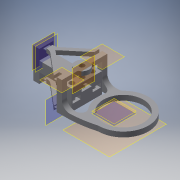
# Autodesk Inventor part: 20_Z-Focus
Saved by Autodesk Inventor 2016 (Build 200138000, 138)
## iProperties
Created: 2016-09-11
Part Number: 20_Z-Focus
Material: Generisch
Document SubType Name: Modeling
Designer: Bene
Density: 1 g/cm^3
Appearance: Vorgabe
Mass: 18.9967 g
Surface Area: 116.758 cm^2
Volume: 18.9967 cm^3
Author: Bene
Autodesk Inventor part; units mm, degrees
ref_plane "YZ Plane" through (0, 0, 0) normal (1, 0, 0) x (0, 1, 0)
ref_plane "XZ Plane" through (0, 0, 0) normal (0, 1, 0) x (-1, 0, 0)
ref_plane "XY Plane" through (0, 0, 0) normal (0, 0, 1) x (1, 0, 0)
ref_plane "Arbeitsebene1" through (0, 0, 0) normal (0, 0, 1) x (1, 0, 0)
ref_plane "Arbeitsebene4" through (-19.17, -30.8266, 13.7758) normal (0, 0, -1) x (-1, 0, 0)
sketch "Skizze3" plane through (-19.17, -30.8266, 13.7758) normal (0, 0, -1) x (-1, 0, 0)
  line L0 (-21.1671, -34.6734) -> (18.8329, -34.6734) construction
  line L1 (23.0052, -34.6734) -> (20.8531, -34.6734) construction
  line L2 (20.8531, -34.6734) -> (20.8531, -31.1843) construction
  line L3 (20.8531, -31.1843) -> (23.0052, -31.1843) construction
  line L4 (23.0052, -31.1843) -> (23.0052, -34.6734) construction
  circle A0 centre (-1.1671, 0.3266) radius 17.5 construction
  line L5 (22.5809, -17.1574) -> (29.5806, -17.1574) construction
  line L6 (29.5806, -17.1574) -> (29.5806, -22.1574) construction
  line L7 (29.5806, -22.1574) -> (28.8232, -22.1574) construction
  line L8 (-0.4194, -22.1574) -> (-0.4194, -17.1574) construction
  line L9 (-0.4194, -22.1574) -> (-21.1671, -22.1574) construction
  line L10 (-21.1671, -22.1574) -> (-21.1671, -17.1574) construction
  line L11 (-21.1671, -17.1574) -> (-0.4194, -17.1574) construction
  line L12 (-0.4194, -17.1574) -> (-0.4194, -22.1574) construction
  line L13 (-21.1671, -17.1574) -> (-17.1671, -17.1574) construction
  line L14 (-17.1671, -17.1574) -> (-17.1671, 0.3266) construction
  line L15 (-17.1671, 0.3266) -> (-21.1671, 0.3266) construction
  line L16 (-21.1671, 0.3266) -> (-21.1671, -17.1574) construction
  line L17 (22.5809, -17.1574) -> (18.5809, -17.1574) construction
  line L18 (18.5809, -10.4487) -> (18.5809, 0.3266) construction
  line L19 (18.5809, 0.3266) -> (22.5809, 0.3266) construction
  line L20 (22.5809, 0.3266) -> (22.5809, -17.1574) construction
  arc A1 (18.5809, -10.4487) -> (-0.4194, -22.1574) centre (-1.1671, 0.3266) ccw construction
  arc A2 (-18.6671, 0.3266) -> (-0.4194, -17.1574) centre (-1.1671, 0.3266) ccw construction
  line L21 (-18.6671, 0.3266) -> (-23.6635, 0.3266) construction
  line L22 (29.5806, -22.1574) -> (-1.9147, -22.1574) construction
  line L23 (29.5806, -17.1574) -> (29.5806, -22.1574)
  arc A3 (-18.6671, 0.3266) -> (16.3329, 0.3266) centre (-1.1671, 0.3266) ccw construction
  line L24 (16.3329, 0.3266) -> (21.3294, 0.3266) construction
  line L25 (-18.6671, 0.3266) -> (-23.6635, 0.3266) construction
  arc A4 (-23.6635, 0.3266) -> (-0.4194, -22.1574) centre (-1.1671, 0.3266) ccw construction
  arc A5 (12.9892, -17.1574) -> (21.3294, 0.3266) centre (-1.1671, 0.3266) ccw construction
  line L26 (-1.9147, -17.1574) -> (-0.4194, -17.1574) construction
  line L27 (28.8232, -22.1574) -> (28.8232, -17.1574)
  line L28 (12.9892, -17.1574) -> (22.5809, -17.1574) construction
  line L29 (28.8232, -17.1574) -> (29.5806, -17.1574)
  line L30 (29.5806, -22.1574) -> (28.8232, -22.1574)
  point P0 (-19.17, 30.8266)
  dimension "d10" = 30
  dimension "d11" = 5
  dimension "d97" = 4
  dimension "d98" = 4
  constraints: 60 end point, 18 point on circle, 13 parallel, 7 perpendicular, 7 point on line, 6 horizontal, 5 centre point, 2 collinear, 2 concentric, 1 coincident
  measures "d10" distance of L8.start L6.end
  measures "d11" distance of L5.end L6.end
  measures "d97" distance of L15.end L14.end
  measures "d98" distance of L18.end L19.end
extrude "Extrusion3" add sketch "Skizze3" along normal blind 5
sketch "Skizze4" plane through (-48.7506, -52.984, 13.7758) normal (-1, 0, 0) x (0, 0, 1)
  line L0 (0, 5) -> (0, 0)
  line L1 (0, 5) -> (-5, 5)
  line L2 (-5, 0) -> (-5, 5)
  line L3 (0, 0) -> (-5, 0)
  line L4 (25, 5) -> (-5, 5)
  line L5 (-5, 5) -> (-5, 0)
  line L6 (-5, 0) -> (25, 0)
  line L7 (25, 0) -> (25, 5)
  line L8 (25, 5) -> (-5, 0) construction
  line L9 (-5, 5) -> (25, 0) construction
  point P0 (-13.7758, 52.984)
  dimension "d17" = 30
  constraints: 20 end point, 2 parallel, 1 horizontal, 1 perpendicular
  measures "d17" distance of L1.end L4.start
extrude "Extrusion4" add sketch "Skizze4" along normal blind 5
ref_plane "Arbeitsebene5" through (-53.7506, -52.984, 13.7758) normal (-1, 0, 0) x (0, 0, 1)
sketch "Skizze5" plane through (-53.7506, -52.984, 13.7758) normal (-1, 0, 0) x (0, 0, 1)
  line L0 (25, 5) -> (-5, 5) projected
  line L1 (-5, 5) -> (-5, 0) projected
  line L2 (-5, 0) -> (25, 0) projected
  line L3 (25, 0) -> (25, 5) projected
  line L4 (25, 5) -> (0, 5) projected
  line L5 (0, 0) -> (25, 0) projected
  line L6 (22, 5) -> (21.3, 5)
  line L7 (21.3, 5) -> (21.3, 0)
  line L8 (21.3, 0) -> (22, 0)
  line L9 (22, 0) -> (22, 5)
  line L10 (-5, 0) -> (25, 0) projected
  line L11 (25, 5) -> (0, 5) projected
  line L12 (-2.7, 0) -> (-2, 0)
  line L13 (-2, 0) -> (-2, 5)
  line L14 (-2, 5) -> (-2.7, 5)
  line L15 (-2.7, 5) -> (-2.7, 0)
  point P0 (-13.7758, 52.984)
  point P1 (-15, 5)
  point P2 (-5, 0)
  point P3 (-5, 5)
  dimension "d20" = 0.7
  dimension "d21" = 0.7
  dimension "d39" = 3
  dimension "d40" = 3
  constraints: 16 end point, 4 parallel, 4 point on line, 2 horizontal, 2 perpendicular
  measures "d20" distance of L8.end L7.end
  measures "d21" distance of L14.end L13.end
  measures "d39" distance between parallel lines of L9 L3
  measures "d40" distance between parallel lines of L1 L13
extrude "Extrusion5" add sketch "Skizze5" along normal blind 3 contours L9 L2 L7 L0 | L13 L2 L15 L0
ref_plane "Arbeitsebene6" through (-48.7506, -52.984, 38.7758) normal (0, 0, 1) x (1, 0, 0)
sketch "Skizze6" plane through (-48.7506, -52.984, 38.7758) normal (0, 0, 1) x (1, 0, 0)
  line L0 (-5, 5) -> (-8, 5) projected
  line L1 (-8, 0) -> (-8, 5) projected
  line L2 (-5, 0) -> (-8, 0) projected
  circle A0 centre (30.7477, 22.484) radius 17.5 projected
  line L3 (30.7477, 22.484) -> (-57.6774, 22.484) construction
  line L4 (30.7477, 22.484) -> (119.1728, 22.484) construction
  line L5 (-5, 0) -> (-8, 0) projected
  line L6 (-8, 0) -> (-34.7954, 22.484)
  line L7 (-8, 0) -> (26.9789, 0) construction
  line L8 (-8, 5) -> (-28.8366, 22.484)
  line L9 (-34.7954, 22.484) -> (-28.8366, 22.484)
  line L10 (-28.8366, 22.484) -> (-34.8366, 22.484)
  line L11 (-34.8366, 22.484) -> (-34.8366, 19.484)
  line L12 (-34.8366, 19.484) -> (-28.8366, 19.484)
  line L13 (-28.8366, 19.484) -> (-28.8366, 22.484)
  line L14 (-5, 5) -> (-5, 0) projected
  point P0 (48.7506, 52.984)
  dimension "d24" = 180
  dimension "d25" = 140
  dimension "d33" = 6
  dimension "d34" = 3
  constraints: 20 end point, 3 horizontal, 2 equal length, 2 parallel, 2 point on line, 1 collinear, 1 perpendicular
  measures "d24" angle of L3 L4
  measures "d25" angle of L7 L6
  measures "d33" distance of L12.end L11.end
  measures "d34" distance of L11.end L10.end
extrude "Extrusion6" add sketch "Skizze6" against normal blind 4 contours L1 L6 L12 L13 L8 | L13 L12 L6 L9 | L12 L11 L10 L6
sketch "Skizze7" plane through (-48.7506, -52.984, 8.7758) normal (0, 0, -1) x (-1, 0, 0)
  line L0 (28.8366, 22.484) -> (8, 5) projected
  line L1 (8, 0) -> (31.2202, 19.484) projected
  line L2 (34.8366, 22.484) -> (28.8366, 22.484) projected
  line L3 (31.2202, 19.484) -> (34.8366, 19.484) projected
  line L4 (34.8366, 19.484) -> (34.8366, 22.484) projected
  line L5 (8, 5) -> (8, 0) projected
  point P0 (48.7506, -52.984)
extrude "Extrusion7" add sketch "Skizze7" against normal blind 4
ref_plane "Arbeitsebene7" through (-83.5872, -33.5, 34.7758) normal (-1, 0, 0) x (0, 0, 1)
sketch "Skizze11" plane through (-83.5872, -33.5, 34.7758) normal (-1, 0, 0) x (0, 0, 1)
  line L0 (4, 3) -> (4, 0) projected
  line L1 (0, 0) -> (0, 3) projected
  line L2 (4, 0) -> (0, 0) projected
  line L3 (-26, 0) -> (-26, 3) projected
  line L4 (-26, 0) -> (-22, 0) projected
  line L5 (-22, 3) -> (-22, 0) projected
  line L6 (4, 0) -> (0, 0) projected
  line L7 (2.45, 6) -> (1.75, 6)
  line L8 (1.75, 6) -> (1.75, 0)
  line L9 (1.75, 0) -> (2.45, 0)
  line L10 (2.45, 0) -> (2.45, 6)
  line L11 (2.45, 6) -> (1.75, 0) construction
  line L12 (1.75, 6) -> (2.45, 0) construction
  line L13 (-26, 0) -> (-22, 0) projected
  line L14 (-23.65, 6) -> (-24.35, 6)
  line L15 (-24.35, 6) -> (-24.35, 0)
  line L16 (-24.35, 0) -> (-23.65, 0)
  line L17 (-23.65, 0) -> (-23.65, 6)
  line L18 (-26, 3) -> (-22, 3) projected
  line L19 (-23.65, 6) -> (-24.35, 0) construction
  line L20 (-24.35, 6) -> (-23.65, 0) construction
  line L21 (4, 3) -> (0, 3) projected
  line L22 (-26, 3) -> (-22, 3) projected
  point P0 (-34.7758, 33.5)
  point P1 (2.1, 3)
  point P2 (-24, 3)
  dimension "d35" = 0.7
  dimension "d36" = 0.7
  constraints: 24 end point, 5 midpoint, 4 parallel, 2 horizontal, 2 perpendicular, 2 point on line
  measures "d35" distance of L9.end L8.end
  measures "d36" distance of L16.end L15.end
extrude "Extrusion9" add sketch "Skizze11" along normal blind 3 contours L21 L8 L7 L10 | L10 L2 L8 L21 | L15 L18 L17 L4 | L15 L14 L17 L18
ref_plane "Arbeitsebene8" through (-86.5872, -33.5, 34.7758) normal (-1, 0, 0) x (0, 0, 1)
sketch "Skizze12" plane through (-86.5872, -33.5, 34.7758) normal (-1, 0, 0) x (0, 0, 1)
  line L0 (2.45, 3) -> (2.45, 0) projected
  line L1 (4, 0) -> (2.45, 0) projected
  line L2 (4, 3) -> (4, 0) projected
  line L3 (-24.35, 0) -> (-24.35, 3) projected
  line L4 (-26, 0) -> (-26, 3) projected
  line L5 (-26, 0) -> (-24.35, 0) projected
  line L6 (4, 6) -> (4, 0) projected
  line L7 (4, 6) -> (-26, 6)
  line L8 (-26, 6) -> (-26, 0)
  line L9 (-26, 0) -> (4, 0)
  line L10 (4, 0) -> (4, 6)
  line L11 (-26, -19.484) -> (-26, 0) projected
  line L12 (4, 10) -> (-26, 10)
  line L13 (-26, 10) -> (-26, -4)
  line L14 (-26, -4) -> (4, -4)
  line L15 (4, -4) -> (4, 10)
  line L16 (4, 10) -> (-26, -4) construction
  line L17 (-26, 10) -> (4, -4) construction
  line L18 (-26, 3) -> (-24.35, 3) projected
  line L19 (4, 3) -> (2.45, 3) projected
  point P0 (-34.7758, 33.5)
  point P1 (-11, 3)
  dimension "d42" = 14
  constraints: 20 end point, 4 parallel, 2 horizontal, 2 midpoint, 2 perpendicular, 2 point on line
  measures "d42" distance of L13.end L12.end
extrude "Extrusion10" add sketch "Skizze12" along normal blind 6
ref_plane "Arbeitsebene9" through (-86.5872, -33.5, 34.7758) normal (1, 0, 0) x (0, 0, -1)
sketch "Skizze21" plane through (-86.5872, -33.5, 34.7758) normal (1, 0, 0) x (0, 0, -1)
  line L0 (-2.45, 0) -> (-2.45, 6) projected
  line L1 (-1.75, 6) -> (-1.75, 0) projected
  line L2 (-1.75, 0) -> (-2.45, 0) projected
  line L3 (23.65, 0) -> (23.65, 6) projected
  line L4 (24.35, 6) -> (24.35, 0) projected
  line L5 (24.35, 0) -> (23.65, 0) projected
  line L6 (26, -4) -> (-4, -4) projected
  line L7 (26, 10) -> (26, -4) projected
  line L8 (-4, 10) -> (26, 10) projected
  line L9 (-4, -4) -> (-4, 10) projected
  line L10 (26, -4) -> (-4, -4) projected
  line L11 (16, 10) -> (6, 10)
  line L12 (6, 10) -> (6, -4)
  line L13 (6, -4) -> (16, -4)
  line L14 (16, -4) -> (16, 10)
  line L15 (16, 10) -> (6, -4) construction
  line L16 (6, 10) -> (16, -4) construction
  line L17 (-2.45, 6) -> (-1.75, 6) projected
  line L18 (23.65, 6) -> (24.35, 6) projected
  point P0 (34.7758, 33.5)
  point P1 (11, 3)
  dimension "d79" = 10
  constraints: 12 end point, 2 midpoint, 2 parallel, 1 horizontal, 1 perpendicular, 1 point on line
  measures "d79" distance of L13.end L12.end
extrude "Extrusion18" add sketch "Skizze21" along normal blind 40 contours L6 L12 L8 L14
ref_plane "Arbeitsebene14" through (-19.17, -30.8266, 15.7758) normal (0, 0, 1) x (1, 0, 0)
sketch "Skizze22" plane through (-19.17, -30.8266, 15.7758) normal (0, 0, 1) x (1, 0, 0)
  circle A0 centre (1.1671, 0.3266) radius 17.5 projected
  line L0 (-18.8329, 35.3266) -> (21.1671, 35.3266) projected
  line L1 (-18.8329, -34.6734) -> (-18.8329, 35.3266) projected
  line L2 (21.1671, -34.6734) -> (-18.8329, -34.6734) projected
  line L3 (21.1671, 35.3266) -> (21.1671, -34.6734) projected
  point P0 (19.17, 30.8266)
extrude "Extrusion19" cut sketch "Skizze22" against normal up to surface (2 mm away)
ref_plane "Arbeitsebene11" through (-48.7506, -13.016, 38.7758) normal (0, 0, 1) x (1, 0, 0)
sketch "Skizze23" plane through (-48.7506, -13.016, 38.7758) normal (0, 0, 1) x (1, 0, 0)
  line L0 (0, 5) -> (0, 0) projected
  line L1 (0, 5) -> (-5, 5) projected
  line L2 (-5, 5) -> (-5, 0) projected
  line L3 (0, 0) -> (-5, 0) projected
  line L4 (0, -39.968) -> (0, -34.968) projected
  line L5 (0, -34.968) -> (-5, -34.968) projected
  line L6 (-5, -39.968) -> (-5, -34.968) projected
  line L7 (0, -39.968) -> (-5, -39.968) projected
  line L8 (-5, 5) -> (0, 5)
  line L9 (0, 5) -> (0, -39.968)
  line L10 (0, -39.968) -> (-5, -39.968)
  line L11 (-5, -39.968) -> (-5, 5)
  circle A0 centre (-2.5, -17.484) radius 7
  line L12 (-37.8366, -24.484) -> (2.1634, -24.484) projected
  point P0 (48.7506, 13.016)
  constraints: 8 end point, 2 parallel, 1 centre point, 1 horizontal, 1 perpendicular, 1 tangent
extrude "Extrusion20" add sketch "Skizze23" against normal blind 4 contours L9 A0 L11 L3 | A0 L9 | L9 A0 L11 | L11 A0 | L9 L12 A0 | A0 L12 L11 | L9 L5 L11 L12
sketch "Skizze24" plane through (-86.5872, -37.5, 18.7758) normal (0, 0, -1) x (-1, 0, 0)
  line L0 (0, 14) -> (0, 0) projected
  line L1 (0, 14) -> (-40, 14) projected
  line L2 (-40, 0) -> (-40, 14) projected
  line L3 (0, 0) -> (-40, 0) projected
  line L4 (-30, -8) -> (-40, -8)
  line L5 (-40, -8) -> (-40, 22)
  line L6 (-40, 22) -> (-30, 22)
  line L7 (-30, 22) -> (-30, -8)
  line L8 (-30, -8) -> (-40, 22) construction
  line L9 (-40, -8) -> (-30, 22) construction
  point P0 (-86.5872, 37.5)
  point P1 (-35, 7)
  dimension "d86" = 30
  constraints: 12 end point, 2 midpoint, 2 parallel, 1 horizontal, 1 perpendicular
  measures "d86" distance of L4.end L5.end
extrude "Extrusion21" add sketch "Skizze24" along normal up to surface (10 mm away) contours L7 L3 L2 L1 | L1 L5 L6 L7 | L7 L4 L5 L3
sketch "Skizze25" plane through (-86.5872, -37.5, 18.7758) normal (0, 0, 1) x (1, 0, 0)
  line L0 (30, 0) -> (40, 0) projected
  line L1 (30, 0) -> (30, -8) projected
  line L2 (30, -8) -> (40, -8) projected
  line L3 (40, -8) -> (40, 0) projected
  line L4 (30, 14) -> (40, 14) projected
  line L5 (40, 14) -> (40, 22) projected
  line L6 (40, 22) -> (30, 22) projected
  line L7 (30, 22) -> (30, 14) projected
  line L8 (30, -8) -> (40, -8) projected
  line L9 (30, -8) -> (40, -8)
  line L10 (40, -8) -> (40, 22)
  line L11 (40, 22) -> (30, 22)
  line L12 (30, 22) -> (30, -8)
  point P0 (86.5872, 37.5)
  constraints: 8 end point, 2 parallel, 1 horizontal, 1 perpendicular
extrude "Extrusion22" add sketch "Skizze25" along normal up to surface (10 mm away) contours L0 L3 L2 L1 | L7 L6 L5 L4
sketch "Skizze26" plane through (-53.7506, -52.984, 38.7758) normal (0, 0, 1) x (1, 0, 0)
  line L0 (0, 0) -> (0, 15.9457) projected
  line L1 (5, 0) -> (0, 0) projected
  line L2 (5, 0) -> (5, 15.9457) projected
  circle A0 centre (2.5, 22.484) radius 2.5
  arc A1 (5, 15.9457) -> (5, 29.0224) centre (2.5, 22.484) ccw projected
  line L3 (5, 29.0224) -> (5, 39.968) projected
  line L4 (5, 39.968) -> (0, 39.968) projected
  line L5 (0, 39.968) -> (0, 29.0224) projected
  arc A2 (0, 29.0224) -> (0, 15.9457) centre (2.5, 22.484) ccw projected
  point P0 (53.7506, 52.984)
  dimension "d91" = 5
  constraints: 1 centre point
  measures "d91" diameter of A0
extrude "Extrusion23" cut sketch "Skizze26" against normal through all contours A0
ref_plane "Arbeitsebene12" through (-46.5872, -33.5, 34.7758) normal (1, 0, 0) x (0, 0, -1)
sketch "Skizze27" plane through (-46.5872, -33.5, 34.7758) normal (1, 0, 0) x (0, 0, -1)
  line L0 (8, -2) -> (14, -2)
  line L1 (14, -2) -> (14, 8)
  line L2 (14, 8) -> (8, 8)
  line L3 (8, 8) -> (8, -2)
  line L4 (8, -2) -> (14, 8) construction
  line L5 (14, -2) -> (8, 8) construction
  point P0 (34.7758, 33.5)
  point P1 (11, 3)
  dimension "d99" = 5
  dimension "d100" = 3
  dimension "d117" = 25.5
  constraints: 12 end point, 2 midpoint, 2 parallel, 1 horizontal, 1 perpendicular
  measures "d99" distance from line of L2 point (11, 3)
  measures "d100" distance from line of L1 point (11, 3)
  measures "d117" distance from line of point (34.776, 33.5) L2
ref_plane "Arbeitsebene13" through (-46.5872, -33.5, 34.7758) normal (1, 0, 0) x (0, 0, -1)
sketch "Skizze29" plane through (-46.5872, -33.5, 34.7758) normal (1, 0, 0) x (0, 0, -1)
  line L0 (6, 18) -> (6, -12) projected
  line L1 (26, -9) -> (6.127, -9) construction
  line L2 (26, -5) -> (6, -5) construction
  line L3 (26, 15) -> (6.127, 15) construction
  line L4 (26, 11) -> (6, 11) construction
  line L5 (15.5291, -11) -> (19.5291, -11) construction
  line L6 (19.5291, -11) -> (19.5291, -3) construction
  line L7 (19.5291, -3) -> (15.5291, -3) construction
  line L8 (15.5291, -3) -> (15.5291, -11) construction
  line L9 (15.5291, -11) -> (19.5291, -3) construction
  line L10 (19.5291, -11) -> (15.5291, -3) construction
  line L11 (15.5291, 17) -> (19.5291, 17)
  line L12 (19.5291, 17) -> (19.5291, 9)
  line L13 (19.5291, 9) -> (15.5291, 9)
  line L14 (15.5291, 9) -> (15.5291, 17)
  line L15 (15.5291, 17) -> (19.5291, 9) construction
  line L16 (19.5291, 17) -> (15.5291, 9) construction
  line L17 (15.5291, -3) -> (19.5291, -3)
  line L18 (19.5291, -3) -> (19.5291, -11)
  line L19 (19.5291, -11) -> (15.5291, -11)
  line L20 (15.5291, -11) -> (15.5291, -3)
  line L21 (15.5291, -3) -> (19.5291, -11) construction
  line L22 (19.5291, -3) -> (15.5291, -11) construction
  line L23 (26, -12) -> (6, -12) projected
  line L24 (26, -12) -> (26, 18) projected
  line L25 (26, 18) -> (6, 18) projected
  point P0 (34.7758, 33.5)
  point P1 (17.5291, -7)
  point P2 (17.5291, 13)
  dimension "d110" = 4
  dimension "d111" = 8
  dimension "d112" = 2
  dimension "d113" = 8
  dimension "d114" = 2
  constraints: 36 end point, 6 midpoint, 6 parallel, 3 horizontal, 3 perpendicular
  measures "d110" distance of L7.end L6.end
  measures "d111" distance of L6.end L5.end
  measures "d112" distance from line of point (17.529, -7) L1
  measures "d113" distance of L11.end L12.end
  measures "d114" distance from line of L4 point (17.529, 13)
extrude "Extrusion26" cut sketch "Skizze29" against normal blind 10 contours L11 L12 L13 L14 | L17 L18 L19 L20
mirror "Spiegeln2" about plane through (-83.5872, -30.5, 38.7758) normal (0, 1, 0) of "Extrusion18", "Extrusion6", "Extrusion5", "Extrusion4", "Extrusion3", "Extrusion7"
extrude "Extrusion27" cut sketch "Skizze27" against normal blind 10
sketch "Skizze30" plane through (-86.5872, -37.5, 28.7758) normal (0, 0, 1) x (1, 0, 0)
  circle A0 centre (35.3366, 7) radius 2.5 projected
  line L0 (40, 1) -> (40, -7) projected
  line L1 (40, 1) -> (30, 1) projected
  line L2 (30, -7) -> (30, 1) projected
  line L3 (40, -7) -> (30, -7) projected
  line L4 (40, 21) -> (40, 13) projected
  line L5 (40, 21) -> (30, 21) projected
  line L6 (30, 13) -> (30, 21) projected
  line L7 (40, 13) -> (30, 13) projected
  circle A1 centre (35.3366, -3) radius 2.5
  line L8 (37.8366, 0.4617) -> (37.8366, -10.484) projected
  circle A2 centre (35.3366, 17) radius 2.5
  point P0 (86.5872, 37.5)
  dimension "d120" = 5
  constraints: 2 centre point, 1 tangent
  measures "d120" diameter of A2
extrude "Extrusion28" cut sketch "Skizze30" against normal blind 40 contours A0 | A1 | A2
sketch "Skizze32" plane through (-46.5872, -45.5, 8.7758) normal (0, 0, -1) x (-1, 0, 0)
  circle A0 centre (4.6634, 5) radius 2.5 construction
  circle A1 centre (4.6634, 15) radius 2.5 construction
  circle A2 centre (4.6634, 25) radius 2.5 construction
  line L0 (0, 0) -> (0, 30) construction
  line L1 (0, 30) -> (10, 30) construction
  line L2 (10, 30) -> (10, 0) construction
  line L3 (10, 0) -> (0, 0) construction
  circle A3 centre (-30, 21.3204) radius 14.8 construction
  line L4 (1.406, 32.484) -> (1.406, 37.484) construction
  line L5 (1.406, -2.484) -> (1.406, -7.484) construction
  line L6 (1.406, 32.484) -> (1.406, 37.484) projected
  line L7 (1.406, 32.484) -> (1.406, 37.484)
  line L8 (1.406, -2.484) -> (1.406, -7.484)
  circle A4 centre (-30, 21.3204) radius 19.8
  circle A5 centre (-30, 21.3204) radius 24.8
  line L9 (1.406, 37.484) -> (-11.191, 37.484)
  line L10 (1.406, 32.484) -> (-7.8547, 32.484)
  line L11 (1.406, -2.484) -> (-23.0437, -2.484)
  arc A6 (-30, -3.4796) -> (1.406, -7.484) centre (-1.3136, 96.3457) ccw
  point P0 (-46.5872, 45.5)
  dimension "d126" = 5
  dimension "d127" = 5
  constraints: 10 end point, 6 point on circle, 3 centre point, 2 parallel, 1 perpendicular
  measures "d126" radial gap between concentric circles of A3 A4
  measures "d127" radial gap between concentric circles of A4 A5
extrude "Extrusion29" add sketch "Skizze32" against normal up to surface (5 mm away)
fillet "Rundung2" radius 5 4 edges at (-35.3962, -8.016, 11.2758) (-38.7325, -13.016, 11.2758) (-16.5872, -48.9796, 11.2758) (-23.5435, -47.984, 11.2758)
fillet "Rundung3" radius 8 2 edges at (-48.7506, -50.484, 13.7758) (-48.7506, -10.516, 13.7758)
fillet "Rundung4" radius 8 6 edges at (-56.5872, -23.5, 24.0113) (-56.5872, -37.5, 24.0113) (-79.9707, -33.5, 10.7758) (-79.9707, -33.5, 36.7758) (-79.9707, -27.5, 36.7758) (-79.9707, -27.5, 10.7758)
sketch "Skizze33" plane through (-46.5872, -45.5, 8.7758) normal (0, 0, -1) x (-1, 0, 0)
  circle A0 centre (4.6634, 5) radius 2.5 projected
  circle A1 centre (4.6634, 25) radius 2.5 projected
  circle A2 centre (4.6634, 15) radius 2.5 projected
  line L0 (0, 0) -> (0, 30) projected
  line L1 (10, 0) -> (0, 0) projected
  arc A3 (10.0627, 1) -> (10, 0) centre (18, 0) ccw projected
  line L2 (10.0627, 1) -> (10, 1) projected
  line L3 (10, 29) -> (10, 1) projected
  line L4 (10.0627, 29) -> (10, 29) projected
  arc A4 (10, 30) -> (10.0627, 29) centre (18, 30) ccw projected
  line L5 (0, 30) -> (10, 30) projected
  line L6 (0, 0) -> (-3, 0)
  line L7 (-3, 0) -> (-3, 30)
  line L8 (-3, 30) -> (0, 30)
  line L9 (0, 30) -> (0, 0)
  point P0 (-46.5872, 45.5)
  dimension "d131" = 13
  constraints: 8 end point, 2 parallel, 1 horizontal, 1 perpendicular
  measures "d131" distance between parallel lines of L7 L3
extrude "Extrusion30" add sketch "Skizze33" against normal up to surface (20 mm away) contours L6 L7 L8 L0
sketch "Skizze36" plane through (-43.5872, -45.5, 8.7758) normal (1, 0, 0) x (0, 0, -1)
  line L0 (-10.4709, 1) -> (-10.4709, 8) projected
  line L1 (-10, 8) -> (-10.4709, 8) projected
  line L2 (-10, 9) -> (-10, 8) projected
  line L3 (-10, 9) -> (-6.4709, 9) projected
  line L4 (-6.4709, 9) -> (-6.4709, 1) projected
  line L5 (-6.4709, 1) -> (-10.4709, 1) projected
  line L6 (-6.4709, 21) -> (-10, 21) projected
  line L7 (-10, 22) -> (-10, 21) projected
  line L8 (-10.4709, 22) -> (-10, 22) projected
  line L9 (-10.4709, 22) -> (-10.4709, 29) projected
  line L10 (-10.4709, 29) -> (-6.4709, 29) projected
  line L11 (-6.4709, 29) -> (-6.4709, 21) projected
  line L12 (-10.4709, 1) -> (-10.4709, 8) projected
  line L13 (-10, 8) -> (-10.4709, 8) projected
  line L14 (-10, 9) -> (-10, 8) projected
  line L15 (-10, 9) -> (-6.4709, 9) projected
  line L16 (-6.4709, 9) -> (-6.4709, 1) projected
  line L17 (-6.4709, 1) -> (-10.4709, 1) projected
  line L18 (-12, 20) -> (-12, 10) projected
  line L19 (-12, 10) -> (-18, 10) projected
  line L20 (-18, 10) -> (-18, 20) projected
  line L21 (-18, 20) -> (-12, 20) projected
  line L22 (-6.4709, 29) -> (-10.4709, 29)
  line L23 (-10.4709, 29) -> (-10.4709, 21)
  line L24 (-10.4709, 21) -> (-6.4709, 21)
  line L25 (-6.4709, 21) -> (-6.4709, 29)
  line L26 (-10, 9) -> (-6.4709, 9) projected
  line L27 (-10.4709, 1) -> (-6.4709, 1)
  line L28 (-6.4709, 1) -> (-6.4709, 9)
  line L29 (-6.4709, 9) -> (-10.4709, 9)
  line L30 (-10.4709, 9) -> (-10.4709, 1)
  point P0 (8.7758, 45.5)
  constraints: 16 end point, 4 parallel, 2 horizontal, 2 perpendicular
extrude "Extrusion31" cut sketch "Skizze36" against normal up to surface (13 mm away)
